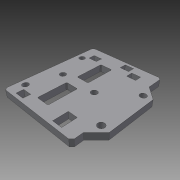
# Autodesk Inventor part: x_motor_top
Saved by Autodesk Inventor 2014 (Build 180170000, 170)
## iProperties
Created: 2013-12-01
Part Number: x_motor_top
Material: Generic
Document SubType Name: Modeling
Designer: buben
Density: 1 g/cm^3
Appearance: Default
Author: buben
Autodesk Inventor part; units mm, degrees
ref_plane "YZ Plane" through (0, 0, 0) normal (1, 0, 0) x (0, 1, 0)
ref_plane "XZ Plane" through (0, 0, 0) normal (0, 1, 0) x (-1, 0, 0)
ref_plane "XY Plane" through (0, 0, 0) normal (0, 0, 1) x (1, 0, 0)
sketch "Sketch1" plane through (0, 0, 0) normal (0, 0, 1) x (1, 0, 0)
  line L0 (0, 0) -> (68, 0)
  line L1 (68, 86) -> (0, 86)
  line L2 (0, 86) -> (0, 0)
  line L3 (68, 71) -> (78, 61)
  line L4 (78, 61) -> (78, 19)
  line L5 (78, 19) -> (68, 9)
  line L6 (68, 0) -> (68, 9)
  line L7 (68, 71) -> (68, 86)
  line L8 (37.5, 83) -> (45.5, 83)
  line L9 (45.5, 83) -> (45.5, 77)
  line L10 (45.5, 77) -> (37.5, 77)
  line L11 (37.5, 77) -> (37.5, 83)
  line L12 (10, 77) -> (18, 77)
  line L13 (18, 77) -> (18, 71)
  line L14 (18, 71) -> (10, 71)
  line L15 (10, 71) -> (10, 77)
  line L16 (10, 9) -> (18, 9)
  line L17 (18, 9) -> (18, 3)
  line L18 (18, 3) -> (10, 3)
  line L19 (10, 3) -> (10, 9)
  line L20 (25, 70) -> (34, 70)
  line L21 (35, 69) -> (35, 46)
  line L22 (34, 45) -> (25, 45)
  line L23 (24, 46) -> (24, 69)
  line L24 (25, 35) -> (34, 35)
  line L25 (35, 34) -> (35, 11)
  line L26 (34, 10) -> (25, 10)
  line L27 (24, 11) -> (24, 34)
  arc A0 (25, 70) -> (24, 69) centre (25, 69) ccw
  arc A1 (35, 69) -> (34, 70) centre (34, 69) ccw
  arc A2 (34, 45) -> (35, 46) centre (34, 46) ccw
  arc A3 (24, 46) -> (25, 45) centre (25, 46) ccw
  arc A4 (25, 35) -> (24, 34) centre (25, 34) ccw
  arc A5 (24, 11) -> (25, 10) centre (25, 11) ccw
  arc A6 (34, 10) -> (35, 11) centre (34, 11) ccw
  arc A7 (35, 34) -> (34, 35) centre (34, 34) ccw
  line L28 (29.5, 70) -> (29.5, 10) construction
  circle A8 centre (71, 60) radius 2.75
  circle A9 centre (71, 20) radius 2.75
  line L29 (48.5, 3) -> (56.5, 3)
  line L30 (56.5, 3) -> (56.5, 9)
  line L31 (56.5, 9) -> (48.5, 9)
  line L32 (48.5, 9) -> (48.5, 3)
  circle A10 centre (6, 13) radius 5 construction
  circle A11 centre (6, 13) radius 2.75
  circle A12 centre (6, 67) radius 5 construction
  circle A13 centre (6, 67) radius 2.75
  line L33 (48.5, 77) -> (56.5, 77)
  line L34 (56.5, 77) -> (56.5, 71)
  line L35 (56.5, 71) -> (48.5, 71)
  line L36 (48.5, 71) -> (48.5, 77)
  line L37 (21, 83) -> (29, 83)
  line L38 (29, 83) -> (29, 77)
  line L39 (29, 77) -> (21, 77)
  line L40 (21, 77) -> (21, 83)
  circle A14 centre (71, 60) radius 5 construction
  circle A15 centre (71, 20) radius 5 construction
  circle A16 centre (14, 40) radius 5 construction
  circle A17 centre (46, 40) radius 5 construction
  circle A18 centre (46, 40) radius 2.75
  circle A19 centre (14, 40) radius 2.75
  line L41 (50, 86) -> (50, 0) construction
  line L42 (55, 86) -> (55, 0) construction
  line L43 (52.5, 86) -> (52.5, 0) construction
  point P0 (78, 40)
  dimension "d1" = 45
  dimension "d2" = 10
  dimension "d3" = 6
  dimension "d4" = 6
  dimension "d5" = 8
  dimension "d6" = 8
  dimension "d7" = 3
  dimension "d8" = 6
  dimension "d9" = 3
  dimension "d12" = 1
  dimension "d13" = 11
  dimension "d14" = 25
  dimension "d15" = 25
  dimension "d16" = 1
  dimension "d17" = 1
  dimension "d18" = 38.5
  dimension "d19" = 5.5
  dimension "d20" = 5.5
  dimension "d21" = 7
  dimension "d23" = 6
  dimension "d24" = 8
  dimension "d25" = 11
  dimension "d26" = 11
  dimension "d27" = 10
  dimension "d28" = 5.5
  dimension "d29" = 5.5
  dimension "d30" = 10
  dimension "d32" = 4
  dimension "d33" = 4
  dimension "d34" = 4
  dimension "d35" = 6
  dimension "d36" = 68
  dimension "d37" = 11.5
  dimension "d38" = 3
  dimension "d39" = 8
  dimension "d40" = 3
  dimension "d41" = 10
  dimension "d42" = 10
  dimension "d43" = 4
  dimension "d44" = 10
  dimension "d45" = 5.5
  dimension "d46" = 10
  dimension "d47" = 5.5
  dimension "d49" = 14
  dimension "d50" = 32
  dimension "d51" = 5
  dimension "d52" = 2.5
  dimension "d53" = 15.5
  dimension "d69" = 86
  constraints: 88 end point, 21 parallel, 20 centre point, 16 point on circle, 16 tangent, 13 collinear, 13 perpendicular, 9 horizontal, 7 equal radius, 6 coincident, 6 point on line, 4 horizontal alignment, 3 midpoint, 1 vertical alignment
  measures "d1" angle of L7 L3
  measures "d2" distance between parallel lines of L7 L4
  measures "d3" distance of L14.end L12.start
  measures "d4" distance of L10.end L8.start
  measures "d5" distance of L12.start L12.end
  measures "d6" distance of L8.start L8.end
  measures "d7" distance between parallel lines of L1 L8
  measures "d8" distance of L18.end L16.start
  measures "d9" distance between parallel lines of L0 L18
  measures "d12" radius of A0
  measures "d13" distance between parallel lines of L21 L23
  measures "d14" distance between parallel lines of L20 L22
  measures "d15" distance between parallel lines of L26 L24
  measures "d16" distance between parallel lines of L20 L14
  measures "d17" distance between parallel lines of L26 L16
  measures "d18" distance between parallel lines of L7 L28
  measures "d19" diameter of A8
  measures "d20" diameter of A9
  measures "d21" distance from line of L4 A9.centre
  measures "d23" distance of L31.end L29.start
  measures "d24" distance of L30.end L31.end
  measures "d25" vertical distance of A9.centre L5.end
  measures "d26" vertical distance of L3.start A8.centre
  measures "d27" diameter of A12
  measures "d28" diameter of A13
  measures "d29" diameter of A11
  measures "d30" diameter of A10
  measures "d32" distance from line of L14 A12.centre
  measures "d33" distance from line of L19 A10.centre
  measures "d34" distance from line of L16 A10.centre
  measures "d35" distance from line of L2 A12.centre
  measures "d36" distance of L0.start L0.end
  measures "d37" distance between parallel lines of L6 L30
  measures "d38" distance between parallel lines of L36 L9
  measures "d39" distance of L38.end L39.end
  measures "d40" distance between parallel lines of L13 L40
  measures "d41" diameter of A14
  measures "d42" diameter of A15
  measures "d43" distance from line of L15 A12.centre
  measures "d44" diameter of A16
  measures "d45" diameter of A19
  measures "d46" diameter of A17
  measures "d47" diameter of A18
  measures "d49" distance from line of L2 A16.centre
  measures "d50" distance from line of L4 A17.centre
  measures "d51" distance between parallel lines of L41 L42
  measures "d52" distance between parallel lines of L41 L43
  measures "d53" distance between parallel lines of L6 L43
  measures "d69" distance of L1.end L0.start
extrude "Extrusion1" add sketch "Sketch1" along normal blind 6
chamfer "Chamfer1" distance 2 angle 45 4 edges at (0, 0, 3) (68, 0, 3) (68, 86, 3) (0, 86, 3)
sketch "Sketch2" plane through (0, 0, 6) normal (0, 0, 1) x (1, 0, 0)
  line L0 (48.5, 9) -> (56.5, 9) projected
  line L1 (68, 2) -> (68, 9) projected
  line L2 (48.5, 15) -> (56.5, 15)
  line L3 (56.5, 15) -> (56.5, 9)
  line L4 (56.5, 9) -> (48.5, 9)
  line L5 (48.5, 9) -> (48.5, 15)
  point P0 (0, 0)
  dimension "d59" = 6
  dimension "d60" = 8
  dimension "d63" = 11.5
  constraints: 8 end point, 2 parallel, 1 collinear, 1 horizontal, 1 perpendicular
  measures "d59" distance of L4.end L2.start
  measures "d60" distance of L2.start L2.end
  measures "d63" distance between parallel lines of L1 L3
extrude "Extrusion2" cut sketch "Sketch2" against normal through all
sketch "Sketch3" plane through (0, 0, 6) normal (0, 0, 1) x (1, 0, 0)
  line L0 (29, 83) -> (29, 77) projected
  line L1 (29, 77) -> (21, 77) projected
  line L2 (21, 77) -> (21, 83) projected
  line L3 (21, 83) -> (29, 83) projected
  point P0 (0, 0)
extrude "Extrusion3" add sketch "Sketch3" against normal blind 6
body "Solid1"
